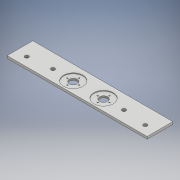
# Autodesk Inventor part: 1021sidemotor
Saved by Autodesk Inventor 2017 (Build 210142000, 142)
## iProperties
Created: 2016-10-15
Part Number: 1021sidemotor
Material: Generic
Document SubType Name: Modeling
Designer: Kevin G
Density: 1 g/cm^3
Appearance: Default
Author: Kevin G
Autodesk Inventor part; units mm, degrees
ref_plane "YZ Plane" through (0, 0, 0) normal (1, 0, 0) x (0, 1, 0)
ref_plane "XZ Plane" through (0, 0, 0) normal (0, 1, 0) x (-1, 0, 0)
ref_plane "XY Plane" through (0, 0, 0) normal (0, 0, 1) x (1, 0, 0)
sketch "Sketch1" plane through (0, 0, 0) normal (0, 0, 1) x (1, 0, 0)
  line L0 (-270.2344, -114.33) -> (-270.2344, -13.08)
  circle A0 centre (-227.9995, -79.405) radius 7.5
  circle A1 centre (-134.4524, -69.88) radius 7.5
  circle A2 centre (-54.3408, -69.88) radius 15.875
  circle A3 centre (-54.3408, -46.8612) radius 2.3813
  circle A4 centre (-31.322, -69.88) radius 2.3813
  circle A5 centre (-77.3595, -69.88) radius 2.3813
  circle A6 centre (-54.3408, -92.8987) radius 2.3813
  line L1 (-270.2344, -13.08) -> (5.175, -13.08)
  line L2 (-270.2344, -114.33) -> (5.1968, -114.33)
  line L3 (280.6281, -114.33) -> (280.6281, -13.08)
  line L4 (280.6281, -13.08) -> (5.175, -13.08)
  line L5 (280.6281, -114.33) -> (5.1968, -114.33)
  circle A7 centre (238.3931, -79.405) radius 7.5
  circle A8 centre (144.846, -69.88) radius 7.5
  circle A9 centre (64.7344, -69.88) radius 15.875
  circle A10 centre (64.7344, -46.8612) radius 2.3813
  circle A11 centre (41.7157, -69.88) radius 2.3813
  circle A12 centre (87.7532, -69.88) radius 2.3813
  circle A13 centre (64.7344, -92.8987) radius 2.3813
  circle A14 centre (64.7344, -69.88) radius 38.1
  circle A15 centre (-54.3408, -69.88) radius 38.1
  point P0 (2, -13.08)
  point P1 (2, -114.33)
  point P2 (-270.2344, -56.825)
  point P3 (-270.2344, -60)
  point P4 (280.6281, -56.825)
  point P5 (280.6281, -60)
  dimension "d4" = 15
  dimension "d7" = 15
  dimension "d9" = 31.75
  dimension "d11" = 4.7625
  dimension "d13" = 4.7625
  dimension "d15" = 23.0188
  dimension "d16" = 4.7625
  dimension "d18" = 4.7625
  dimension "d25" = 550.8625
  dimension "d50" = 23.0188
  dimension "d51" = 23.0188
  dimension "d52" = 23.0188
  dimension "d53" = 80.1116
  dimension "d54" = 93.5471
  dimension "d56" = 119.0752
  dimension "d57" = 80.1116
  dimension "d60" = 93.5471
  dimension "d61" = 76.2
  dimension "d62" = 76.2
  constraints: 16 centre point, 12 end point, 6 point on line, 2 coincident, 1 horizontal
  measures "d4" diameter of A0
  measures "d7" diameter of A1
  measures "d9" diameter of A2
  measures "d11" diameter of A3
  measures "d13" diameter of A4
  measures "d15" distance of A2.centre A5.centre
  measures "d16" diameter of A5
  measures "d18" diameter of A6
  measures "d25" distance between parallel lines of L0 L3
  measures "d50" distance of A3.centre A2.centre
  measures "d51" distance of A4.centre A2.centre
  measures "d52" distance of A2.centre A6.centre
  measures "d53" distance of A2.centre A1.centre
  measures "d54" horizontal distance of A0.centre A1.centre
  measures "d56" distance of A9.centre A2.centre
  measures "d57" distance of A8.centre A9.centre
  measures "d60" horizontal distance of A7.centre A8.centre
  measures "d61" diameter of A14
  measures "d62" diameter of A15
extrude "Extrusion3" add sketch "Sketch1" along normal blind 9.525 contours L0 L1 L4 L3 L5 L2 | A14 | A15
sketch "Sketch4" plane through (0, 0, 9.525) normal (0, 0, 1) x (1, 0, 0)
  line L0 (-270.2344, -114.33) -> (-270.2344, -13.08)
  circle A0 centre (-227.9995, -79.405) radius 7.5
  circle A1 centre (-134.4524, -69.88) radius 7.5
  circle A2 centre (-54.3408, -69.88) radius 15.875
  circle A3 centre (-54.3408, -46.8612) radius 2.3813
  circle A4 centre (-31.322, -69.88) radius 2.3813
  circle A5 centre (-77.3595, -69.88) radius 2.3813
  circle A6 centre (-54.3408, -92.8987) radius 2.3813
  line L1 (-270.2344, -13.08) -> (5.175, -13.08)
  line L2 (-270.2344, -114.33) -> (5.1968, -114.33)
  line L3 (280.6281, -114.33) -> (5.1968, -114.33)
  line L4 (280.6281, -13.08) -> (5.175, -13.08)
  line L5 (280.6281, -114.33) -> (280.6281, -13.08)
  circle A7 centre (238.3931, -79.405) radius 7.5
  circle A8 centre (144.846, -69.88) radius 7.5
  circle A9 centre (64.7344, -69.88) radius 15.875
  circle A10 centre (64.7344, -46.8612) radius 2.3813
  circle A11 centre (41.7157, -69.88) radius 2.3813
  circle A12 centre (64.7344, -92.8987) radius 2.3813
  circle A13 centre (87.7532, -69.88) radius 2.3813
  circle A14 centre (64.7344, -69.88) radius 38.1
  circle A15 centre (-54.3408, -69.88) radius 38.1
  point P0 (0, 0)
  point P1 (2, -13.08)
  point P2 (2, -114.33)
  point P3 (-270.2344, -56.825)
  point P4 (-270.2344, -60)
  point P5 (280.6281, -56.825)
  point P6 (280.6281, -60)
  dimension "d67" = 15
  dimension "d68" = 15
  dimension "d69" = 31.75
  dimension "d70" = 4.7625
  dimension "d71" = 4.7625
  dimension "d72" = 23.0188
  dimension "d73" = 4.7625
  dimension "d74" = 4.7625
  dimension "d75" = 550.8625
  dimension "d76" = 23.0188
  dimension "d77" = 23.0188
  dimension "d78" = 23.0188
  dimension "d79" = 80.1116
  dimension "d80" = 93.5471
  dimension "d81" = 119.0752
  dimension "d82" = 80.1116
  dimension "d83" = 93.5471
  dimension "d84" = 76.2
  dimension "d85" = 76.2
  constraints: 16 centre point, 12 end point, 6 point on line, 2 coincident, 1 horizontal
  measures "d67" diameter of A0
  measures "d68" diameter of A1
  measures "d69" diameter of A2
  measures "d70" diameter of A3
  measures "d71" diameter of A4
  measures "d72" distance of A2.centre A5.centre
  measures "d73" diameter of A5
  measures "d74" diameter of A6
  measures "d75" distance between parallel lines of L0 L5
  measures "d76" distance of A3.centre A2.centre
  measures "d77" distance of A4.centre A2.centre
  measures "d78" distance of A2.centre A6.centre
  measures "d79" distance of A2.centre A1.centre
  measures "d80" horizontal distance of A0.centre A1.centre
  measures "d81" distance of A9.centre A2.centre
  measures "d82" distance of A8.centre A9.centre
  measures "d83" horizontal distance of A7.centre A8.centre
  measures "d84" diameter of A14
  measures "d85" diameter of A15
emboss "Emboss3" sketch "Sketch4" operation cut depth 3 direction (0, 0, -1) contours A14 | A15
body "Solid3"
